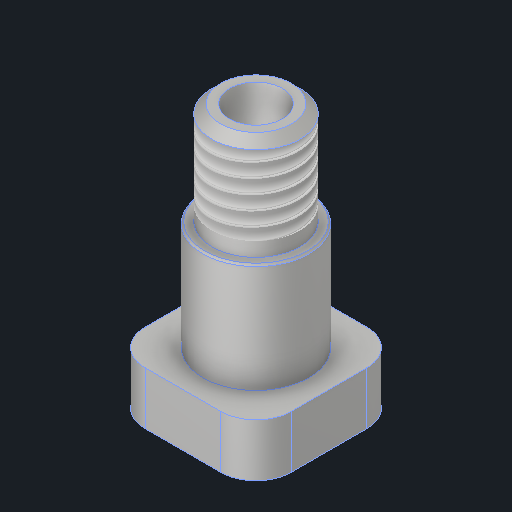
# Autodesk Inventor part: Radadapter
Saved by Autodesk Inventor 2026.1 (Build 301233000, 233)
## iProperties
Part Number: Radadapter
Material: Aluminium 6061
Document SubType Name: Modeling
Designer: rYan
Mass: 1.61876 g
Surface Area: 6.69144 cm^2
Volume: 0.59954 cm^3
Density: 2.7 g/cm^3
Appearance: Aluminium - flach
Author: rYan
Autodesk Inventor part; units mm, degrees
ref_plane "YZ Plane" through (0, 0, 0) normal (1, 0, 0) x (0, 1, 0)
ref_plane "XZ Plane" through (0, 0, 0) normal (0, 1, 0) x (-1, 0, 0)
ref_plane "XY Plane" through (0, 0, 0) normal (0, 0, 1) x (1, 0, 0)
sketch "Skizze1" plane through (0, 0, 0) normal (0, 0, 1) x (1, 0, 0)
  line L0 (-2.15, 4.15) -> (2.15, 4.15)
  line L1 (4.15, 2.15) -> (4.15, -2.15)
  line L2 (2.15, -4.15) -> (-2.15, -4.15)
  line L3 (-4.15, -2.15) -> (-4.15, 2.15)
  arc A0 (-2.15, 4.15) -> (-4.15, 2.15) centre (-2.15, 2.15) ccw
  arc A1 (4.15, 2.15) -> (2.15, 4.15) centre (2.15, 2.15) ccw
  arc A2 (2.15, -4.15) -> (4.15, -2.15) centre (2.15, -2.15) ccw
  arc A3 (-4.15, -2.15) -> (-2.15, -4.15) centre (-2.15, -2.15) ccw
  line L4 (-2.15, 2.15) -> (2.15, -2.15) construction
  line L5 (2.15, 2.15) -> (-2.15, -2.15) construction
  point P0 (0, 0)
  dimension "d0" = 2
  dimension "d1" = 8.3
  constraints: 12 end point, 8 point on circle, 8 tangent, 4 centre point, 3 equal radius, 2 midpoint, 2 parallel, 2 perpendicular, 1 horizontal
  measures "d0" radius of A0
  measures "d1" distance between parallel lines of L2 L0
extrude "Extrusion1" add sketch "Skizze1" along normal blind 3
sketch "Skizze2" plane through (0, 0, 3) normal (0, 0, 1) x (1, 0, 0)
  circle A0 centre (0, 0) radius 2.5
  circle A1 centre (0, 0) radius 3
  dimension "d4" = 5
  dimension "d22" = 6
  constraints: 2 centre point, 2 coincident
  measures "d4" diameter of A0
  measures "d22" diameter of A1
extrude "Extrusion2" add sketch "Skizze2" along normal blind 12 contours A0
sketch "Skizze3" plane through (0, 0, 15) normal (0, 0, 1) x (1, 0, 0)
  point P0 (0, 0)
  point P1 (0, 0)
  constraints: 1 coincident
hole "Bohrung1" at (0, 0, 15) direction (0, 0, -1) diameter 3 end through all
chamfer "Fase1" distance 0.5 angle 45 1 edges at (-2.5, 0, 15)
thread "Gewinde2" size "M5x0.8" class "6g" standard "ISO Metric profile" length 4.5
extrude "Extrusion3" add sketch "Skizze2" along normal blind 6.2
sketch "Skizze4" plane through (0, 0, 0) normal (0, 0, -1) x (-1, 0, 0)
  point P0 (0, 0)
  point P1 (0, 0)
  constraints: 1 coincident
hole "Bohrung2" [suppressed]
chamfer "Fasen2" distance 0.1 angle 45 2 edges at (-3, 0, 9.2) (0, 1.5, 0)
